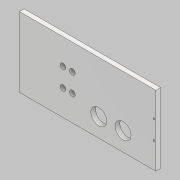
# Autodesk Inventor part: CW001
Saved by Autodesk Inventor 2017 (Build 210142000, 142)
## iProperties
Created: 2017-05-22
Part Number: CW001
Material: ABS Plastic
Document SubType Name: Modeling
Designer: zallen
Density: 1.06 g/cm^3
Appearance: CR White
Author: zallen
Autodesk Inventor part; units mm, degrees
ref_plane "YZ Plane" through (0, 0, 0) normal (1, 0, 0) x (0, 1, 0)
ref_plane "XZ Plane" through (0, 0, 0) normal (0, 1, 0) x (-1, 0, 0)
ref_plane "XY Plane" through (0, 0, 0) normal (0, 0, 1) x (1, 0, 0)
sketch "Sketch1" plane through (0, 0, 0) normal (0, 0, 1) x (1, 0, 0)
  line L0 (0, 0) -> (145.9214, 0)
  line L1 (145.9214, 0) -> (145.9214, 5)
  line L2 (145.9214, 5) -> (0, 5)
  line L3 (0, 5) -> (0, 0)
  dimension "d0" = 145.9214
  dimension "d1" = 5
  constraints: 8 end point, 2 parallel, 1 horizontal, 1 perpendicular
  measures "d0" distance of L2.end L1.end
  measures "d1" distance of L1.end L0.end
extrude "Extrusion1" add sketch "Sketch1" along normal blind 75
sketch "Sketch2" plane through (0, 0, 0) normal (0, -1, 0) x (1, 0, 0)
  circle A0 centre (46.6338, 27.5) radius 3
  line L0 (0, 0) -> (145.9214, 0) projected
  line L1 (0, 0) -> (0, 75) projected
  circle A1 centre (46.6338, 47.5) radius 3
  circle A2 centre (56.6338, 47.5) radius 3
  circle A3 centre (56.6338, 27.5) radius 3
  dimension "d4" = 6
  dimension "d5" = 27.5
  dimension "d6" = 46.6338
  dimension "d7" = 6
  dimension "d8" = 20
  dimension "d9" = 6
  dimension "d10" = 6
  dimension "d11" = 10
  constraints: 4 centre point, 2 horizontal alignment, 2 vertical alignment
  measures "d4" diameter of A0
  measures "d5" distance from line of L0 A0.centre
  measures "d6" distance from line of L1 A0.centre
  measures "d7" diameter of A1
  measures "d8" distance of A0.centre A1.centre
  measures "d9" diameter of A2
  measures "d10" diameter of A3
  measures "d11" distance of A2.centre A1.centre
extrude "Extrusion2" cut sketch "Sketch2" against normal through all
sketch "Sketch3" plane through (0, 0, 0) normal (0, -1, 0) x (1, 0, 0)
  circle A0 centre (46.6338, 27.5) radius 3 projected
  circle A1 centre (143.9214, 27.5) radius 1
  circle A2 centre (143.9214, 47.5) radius 1
  circle A3 centre (46.6338, 47.5) radius 3 projected
  line L0 (145.9214, 0) -> (145.9214, 75) projected
  point P0 (0, 0)
  dimension "d22" = 2
  dimension "d23" = 2
  dimension "d24" = 2
  constraints: 2 centre point, 2 horizontal alignment, 1 vertical alignment
  measures "d22" diameter of A1
  measures "d23" diameter of A2
  measures "d24" distance from line of L0 A1.centre
extrude "Extrusion3" cut sketch "Sketch3" against normal through all contours A1 | A2
thread "Thread7" size "M2x0.4" class "6H" standard "ANSI Metric M Profile" full length
thread "Thread8" size "M2x0.4" class "6H" standard "ANSI Metric M Profile" full length
sketch "Sketch4" plane through (0, 0, 0) normal (0, -1, 0) x (1, 0, 0)
  circle A0 centre (110.9214, 20) radius 8.5
  line L0 (145.9214, 0) -> (145.9214, 75) projected
  line L1 (0, 75) -> (145.9214, 75) projected
  circle A1 centre (84.9214, 20) radius 8.5
  point P0 (0, 0)
  dimension "d35" = 17
  dimension "d36" = 35
  dimension "d38" = 17
  dimension "d39" = 26
  dimension "d42" = 20
  constraints: 2 centre point, 1 horizontal alignment
  measures "d35" diameter of A0
  measures "d36" distance from line of L0 A0.centre
  measures "d38" diameter of A1
  measures "d39" distance of A0.centre A1.centre
  measures "d42" vertical distance of L0.start A0.centre
extrude "Extrusion4" cut sketch "Sketch4" against normal through all
body "Solid1"
